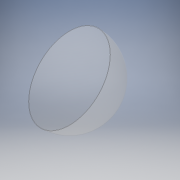
# Autodesk Inventor part: Covering
Saved by Autodesk Inventor 2018 (Build 220112000, 112)
## iProperties
Created: 2019-05-31
Part Number: Covering
Material: Generic
Document SubType Name: Modeling
Designer: ch1180245
Density: 1 g/cm^3
Appearance: Default
Author: ch1180245
Autodesk Inventor part; units mm, degrees
ref_plane "YZ Plane" through (0, 0, 0) normal (1, 0, 0) x (0, 1, 0)
ref_plane "XZ Plane" through (0, 0, 0) normal (0, 1, 0) x (-1, 0, 0)
ref_plane "XY Plane" through (0, 0, 0) normal (0, 0, 1) x (1, 0, 0)
sketch "Sketch1" plane through (0, 0, 0) normal (1, 0, 0) x (0, 1, 0)
  arc A0 (-850, 0) -> (850, 0) centre (0, 0) ccw
  line L0 (850, 0) -> (-850, 0)
  arc A1 (-840, 0) -> (840, 0) centre (0, 0) ccw
  line L1 (-1190, 0) -> (1190, 0) projected
  dimension "d0" = 1700
  dimension "d1" = 840
  constraints: 4 point on circle, 2 centre point, 2 coincident, 2 end point, 2 point on line, 1 horizontal
  measures "d0" diameter of A0
  measures "d1" radius of A1
revolve "Revolution1" add sketch "Sketch1" angle 180 about axis through (0, -10, 0) along (0, -1, 0) contours L0 A1 A0
body "Solid1"
